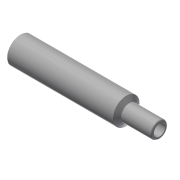
# Autodesk Inventor part: Pieza6
Saved by Autodesk Inventor 2021 (Build 250183000, 183)
## iProperties
Created: 2013-06-02
Part Number: Pieza6
Material: Acero
Document SubType Name: Modeling
Designer: BRAYAN
Density: 1 g/cm^3
Appearance: Steel
Author: BRAYAN
Autodesk Inventor part; units mm, degrees
ref_plane "YZ Plane" through (0, 0, 0) normal (1, 0, 0) x (0, 1, 0)
ref_plane "XZ Plane" through (0, 0, 0) normal (0, 1, 0) x (-1, 0, 0)
ref_plane "XY Plane" through (0, 0, 0) normal (0, 0, 1) x (1, 0, 0)
sketch "Boceto1" plane through (0, 0, 0) normal (0, 0, 1) x (1, 0, 0)
  line L0 (0, 0) -> (0, 17.526)
  line L1 (0, 17.526) -> (140, 17.526)
  line L2 (140, 17.526) -> (144, 11)
  line L3 (144, 11) -> (184, 11)
  line L4 (184, 11) -> (184, 0)
  line L5 (144, 7.474) -> (184, 7.474)
  line L6 (184, 0) -> (0, 0)
  line L7 (0, 17.526) -> (0, 14)
  line L8 (0, 14) -> (140, 14)
  line L9 (144, 7.474) -> (140, 14)
  point P0 (0, 11.6562)
  dimension "d5" = 140
  dimension "d9" = 40
  dimension "d13" = 17.526
  dimension "d14" = 14
  constraints: 20 end point, 4 perpendicular, 3 point on line, 2 parallel
  measures "d5" distance of L0.end L1.end
  measures "d9" distance of L2.end L3.end
  measures "d13" distance between parallel lines of L1 L6
  measures "d14" distance between parallel lines of L8 L6
revolve "Revolución2" add sketch "Boceto1" angle 360 about axis through (184, 0, 0) along (-1, 0, 0) contours L0 L1 L2 L3 L4 L5 L9 L8
fillet "Empalme2" radius 2 1 edges at (184, -11, 0)
equation "\"d13\" = 0.5 * DintTub"
equation "\"d14\" = 0.5 * DIntTubTen"
equation "\"DintTub\" = 35.052"
equation "\"DIntTubTen\" = 28"
